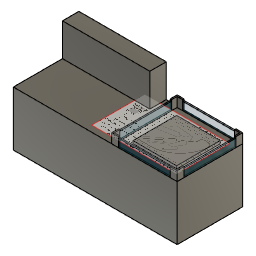
CTTM v2 (Autodesk Fusion 360 design; units mm, degrees)
Autodesk Fusion 360 part; units mm, degrees
sketch "Sketch1" plane through (0, 0, 0) normal (0, 0, 1) x (1, 0, 0)
  line L0 (0, 0) -> (-762, 0)
  line L1 (-762, 0) -> (-762, -304.8)
  line L2 (-762, -304.8) -> (0, -304.8)
  line L3 (0, -304.8) -> (0, 0)
  line L4 (0, -304.8) -> (-304.8, -304.8)
  line L5 (-304.8, -304.8) -> (-304.8, 0)
  line L6 (-304.8, 0) -> (0, 0)
  line L7 (0, 0) -> (0, -304.8)
  line L8 (-6.35, -6.35) -> (-298.45, -6.35)
  line L9 (-298.45, -6.35) -> (-298.45, -298.45)
  line L10 (-298.45, -298.45) -> (-6.35, -298.45)
  line L11 (-6.35, -298.45) -> (-6.35, -6.35)
  line L12 (-304.8, -6.35) -> (-304.8, 0)
  line L13 (-304.8, 0) -> (-298.45, 0)
  line L14 (0, -6.35) -> (0, 0)
  line L15 (0, 0) -> (-6.35, 0)
  line L16 (-6.35, -6.35) -> (-31.75, -6.35)
  line L17 (-31.75, -6.35) -> (-31.75, 0)
  line L18 (-31.75, 0) -> (-6.35, 0)
  line L19 (0, -6.35) -> (0, -31.75)
  line L20 (0, -31.75) -> (-6.35, -31.75)
  line L21 (-6.35, -31.75) -> (-6.35, -6.35)
  line L22 (-298.45, -6.35) -> (-298.45, -31.75)
  line L23 (-298.45, -31.75) -> (-304.8, -31.75)
  line L24 (-304.8, -31.75) -> (-304.8, -6.35)
  line L25 (-298.45, -6.35) -> (-273.05, -6.35)
  line L26 (-273.05, -6.35) -> (-273.05, 0)
  line L27 (-273.05, 0) -> (-298.45, 0)
  line L28 (-298.45, -298.45) -> (-273.05, -298.45)
  line L29 (-273.05, -298.45) -> (-273.05, -304.8)
  line L30 (-273.05, -304.8) -> (-298.45, -304.8)
  line L31 (-304.8, -298.45) -> (-304.8, -273.05)
  line L32 (-304.8, -273.05) -> (-298.45, -273.05)
  line L33 (-298.45, -273.05) -> (-298.45, -298.45)
  line L34 (0, -298.45) -> (0, -273.05)
  line L35 (0, -273.05) -> (-6.35, -273.05)
  line L36 (-6.35, -273.05) -> (-6.35, -298.45)
  line L37 (-6.7592, -298.45) -> (-32.1592, -298.45)
  line L38 (-32.1592, -298.45) -> (-32.1592, -304.8)
  line L39 (-32.1592, -304.8) -> (-6.7592, -304.8)
  point P0 (-152.4, -152.4)
  dimension "d1" = 762
  dimension "d2" = 304.8
  dimension "d3" = 304.8
  dimension "d4" = 292.1
  dimension "d5" = 292.1
  dimension "d6" = 25.4
  dimension "d7" = 25.4
  dimension "d8" = 25.4
  dimension "d9" = 25.4
  dimension "d10" = 25.4
  dimension "d11" = 25.4
  dimension "d12" = 25.4
  dimension "d13" = 25.4
  constraint horizontal L0
  constraint vertical L1
  constraint horizontal L2
  constraint vertical L3
  constraint coincident L0.start L3.end
  constraint horizontal L4
  constraint vertical L5
  constraint horizontal L6
  constraint vertical L7
  constraint horizontal L8
  constraint perpendicular L8 L9
  constraint parallel L8 L10
  constraint parallel L9 L11
  constraint vertical L12
  constraint horizontal L13
  constraint vertical L14
  constraint horizontal L15
  constraint horizontal L16
  constraint vertical L17
  constraint horizontal L18
  constraint vertical L19
  constraint horizontal L20
  constraint vertical L21
  constraint vertical L22
  constraint horizontal L23
  constraint vertical L24
  constraint horizontal L25
  constraint vertical L26
  constraint horizontal L27
  constraint horizontal L28
  constraint vertical L29
  constraint horizontal L30
  constraint vertical L31
  constraint horizontal L32
  constraint vertical L33
  constraint vertical L34
  constraint horizontal L35
  constraint vertical L36
  constraint horizontal L37
  constraint vertical L38
  constraint horizontal L39
  constraint coincident L10 L37.start
  measures "d1" distance of L0.start L0.end
  measures "d2" distance of L0.start L2.end
  measures "d3" distance of L2.end L4.end
  measures "d4" distance of L9.end L10.end
  measures "d5" distance of L8.end L9.end
  measures "d6" distance of L8.start L16.end
  measures "d7" distance of L8.start L20.end
  measures "d8" distance of L12.start L23.end
  measures "d9" distance of L8.end L25.end
  measures "d10" distance of L9.end L28.end
  measures "d11" distance of L9.end L32.end
  measures "d12" distance of L10.end L35.end
  measures "d13" distance of L37.start L37.end
extrude "Extrude1" add sketch "Sketch1" against normal blind 254 makes body 1
extrude "Extrude1'" add sketch "Sketch1" along normal blind 38.1 separate body contours L0 L6 L8 L17 L26 | L3 L7 L11 L20 L35 | L5 L9 L23 L32 | L2 L4 L10 L29 L38 makes body 2 at (0, -192.6167, 12.7) makes body 3 at (-304.8, -192.6167, 12.7) makes body 4 at (-112.1833, -6.35, 12.7) makes body 5 at (-192.7531, -304.8, 12.7) in component "Water Bath Glass"
copy_body "Body->Comp1" bodies 1 removing the originals makes body 6 in component "Component"
extrude "Extrude1''" add sketch "Sketch1" along normal blind 44.45 separate body contours L0 L3 L6 L7 L8 L11 L14 L15 L16 L17 L18 L19 L20 L21 | L0 L5 L6 L8 L9 L12 L13 L22 L23 L24 L25 L26 L27 | L2 L3 L4 L7 L10 L11 L34 L35 L36 L37 L38 L39 | L2 L4 L5 L9 L10 L28 L29 L30 L31 L32 L33 makes body 7 at (-283.6333, 0, 29.6333) makes body 8 at (-21.4395, -304.8, 14.8167) makes body 9 at (-21.1667, 0, 14.8167) makes body 10 at (-294.2167, -304.8, 29.6333) in component "Component'"
sketch "Sketch2" plane through (0, 0, 0) normal (0, 0, 1) x (-1, 0, 0)
  line L0 (762, 304.8) -> (0, 304.8)
  line L1 (0, 304.8) -> (0, 0)
  line L2 (0, 0) -> (762, 0)
  line L3 (762, 0) -> (762, 304.8)
  line L4 (298.45, 6.35) -> (273.05, 6.35)
  line L5 (273.05, 6.35) -> (273.05, 0)
  line L6 (273.05, 0) -> (304.8, 0)
  line L7 (304.8, 0) -> (304.8, 31.75)
  line L8 (304.8, 31.75) -> (298.45, 31.75)
  line L9 (298.45, 31.75) -> (298.45, 6.35)
  line L10 (298.45, 31.75) -> (304.8, 31.75)
  line L11 (304.8, 31.75) -> (304.8, 273.05)
  line L12 (304.8, 273.05) -> (298.45, 273.05)
  line L13 (298.45, 273.05) -> (298.45, 31.75)
  line L14 (298.45, 273.05) -> (304.8, 273.05)
  line L15 (304.8, 273.05) -> (304.8, 304.8)
  line L16 (304.8, 304.8) -> (273.05, 304.8)
  line L17 (273.05, 304.8) -> (273.05, 298.45)
  line L18 (273.05, 298.45) -> (298.45, 298.45)
  line L19 (298.45, 298.45) -> (298.45, 273.05)
  line L20 (762, 0) -> (355.6, 0)
  line L21 (355.6, 0) -> (355.6, 76.2)
  line L22 (355.6, 76.2) -> (762, 76.2)
  line L23 (762, 76.2) -> (762, 0)
  dimension "d20" = 406.4
  dimension "d21" = 76.2
  constraint horizontal L20
  constraint vertical L21
  constraint horizontal L22
  constraint vertical L23
  constraint coincident L2.end L3.start
  measures "d20" distance of L2.end L20.end
  measures "d21" distance of L2.end L22.end
extrude "Extrude1'''" add sketch "Sketch2" along normal blind 152.4 contours L2 L3 L20 L21 L22 L23 bodies 6 in component "Component"
sketch "Sketch3" plane through (0, 0, 0) normal (0, 0, 1) x (-1, 0, 0)
  line L0 (355.6, 0) -> (355.6, 76.2)
  line L1 (355.6, 76.2) -> (762, 76.2)
  line L2 (762, 76.2) -> (762, 304.8)
  line L3 (762, 304.8) -> (0, 304.8)
  line L4 (0, 304.8) -> (0, 0)
  line L5 (0, 0) -> (355.6, 0)
  line L6 (31.75, 6.35) -> (31.75, 0)
  line L7 (31.75, 0) -> (273.05, 0)
  line L8 (273.05, 0) -> (273.05, 6.35)
  line L9 (273.05, 6.35) -> (31.75, 6.35)
  line L10 (273.05, 298.45) -> (273.05, 304.8)
  line L11 (273.05, 304.8) -> (32.1592, 304.8)
  line L12 (32.1592, 304.8) -> (32.1592, 298.45)
  line L13 (32.1592, 298.45) -> (273.05, 298.45)
  line L14 (0, 31.75) -> (6.35, 31.75)
  line L15 (6.35, 31.75) -> (6.35, 273.05)
  line L16 (6.35, 273.05) -> (0, 273.05)
  line L17 (0, 273.05) -> (0, 31.75)
  line L18 (298.45, 31.75) -> (304.8, 31.75)
  line L19 (304.8, 31.75) -> (304.8, 273.05)
  line L20 (304.8, 273.05) -> (298.45, 273.05)
  line L21 (298.45, 273.05) -> (298.45, 31.75)
  line L22 (762, 76.2) -> (355.6, 76.2)
  line L23 (355.6, 76.2) -> (355.6, 0)
  line L24 (355.6, 0) -> (762, 0)
  line L25 (762, 0) -> (762, 76.2)
  line L26 (50.8, 50.8) -> (254, 50.8)
  line L27 (254, 50.8) -> (254, 254)
  line L28 (254, 254) -> (50.8, 254)
  line L29 (50.8, 254) -> (50.8, 50.8)
  line L30 (50.8, 50.8) -> (254, 254) construction
  line L31 (254, 50.8) -> (50.8, 254) construction
  point P0 (152.4, 152.4)
  dimension "d24" = 203.2
  dimension "d25" = 203.2
  constraint horizontal L26
  constraint perpendicular L26 L27
  constraint parallel L26 L28
  constraint parallel L27 L29
  constraint coincident L30 P0
  constraint coincident L31 P0
  measures "d24" distance of L27.end L28.end
  measures "d25" distance of L26.end L27.end
extrude "Extrude1''''" add sketch "Sketch3" along normal blind 12.7 separate body contours L26 L27 L28 L29 makes body 11 in component "Component''"
component "Water Bath Glass" placed x (1, 0, 0) y (0, 1, 0) z (0, 0, 1) at (0, 0, 0)
component "Component" placed x (1, 0, 0) y (0, 1, 0) z (0, 0, 1) at (0, 0, 0)
component "Component'" placed x (1, 0, 0) y (0, 1, 0) z (0, 0, 1) at (0, 0, 0)
component "Component''" placed x (1, 0, 0) y (0, 1, 0) z (0, 0, 1) at (0, 0, 0)
